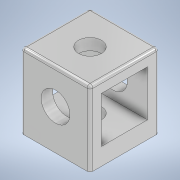
# Autodesk Inventor part: Kutup Aki
Saved by Autodesk Inventor 2021 (Build 250183000, 183)
## iProperties
Created: 2023-04-01
Part Number: Kutup Aki
Material: Iron, Cast
Document SubType Name: Modeling
Designer: user
Density: 7.15 g/cm^3
Appearance: Aluminum - Polished
Author: user
Autodesk Inventor part; units mm, degrees
ref_plane "YZ Plane" through (0, 0, 0) normal (1, 0, 0) x (0, 1, 0)
ref_plane "XZ Plane" through (0, 0, 0) normal (0, 1, 0) x (-1, 0, 0)
ref_plane "XY Plane" through (0, 0, 0) normal (0, 0, 1) x (1, 0, 0)
sketch "Sketch1" plane through (0, 0, 0) normal (0, 1, 0) x (-1, 0, 0)
  line L0 (6, -6) -> (-6, -6)
  line L1 (-6, -6) -> (-6, 6)
  line L2 (-6, 6) -> (6, 6)
  line L3 (6, 6) -> (6, -6)
  line L4 (6, -6) -> (-6, 6) construction
  line L5 (-6, -6) -> (6, 6) construction
  point P0 (0, 0)
  dimension "d0" = 12
  dimension "d1" = 12
  constraints: 12 end point, 2 midpoint, 2 parallel, 1 horizontal, 1 perpendicular
  measures "d0" distance of L1.end L2.end
  measures "d1" distance of L0.end L1.end
extrude "Extrusion1" add sketch "Sketch1" along normal blind 13
sketch "Sketch2" plane through (6, 0, 6) normal (1, 0, 0) x (0, 0, -1)
  line L0 (0, 0) -> (0, 13) projected
  line L1 (0, 13) -> (12, 13) projected
  line L2 (12, 13) -> (12, 0) projected
  line L3 (12, 0) -> (0, 0) projected
  line L4 (10, 11) -> (2, 11)
  line L5 (2, 11) -> (2, 2)
  line L6 (2, 2) -> (10, 2)
  line L7 (10, 2) -> (10, 11)
  line L8 (2, 11) -> (10, 11)
  line L9 (10, 11) -> (10, 3)
  line L10 (10, 3) -> (2, 3)
  line L11 (2, 3) -> (2, 11)
  point P0 (6, 0)
  dimension "d4" = 2
  dimension "d5" = 8
  dimension "d6" = 8
  constraints: 16 end point, 2 parallel, 1 horizontal, 1 perpendicular, 3 other
  measures "d4" distance between parallel lines of L1 L4
  measures "d5" distance of L9.end L10.end
  measures "d6" distance of L8.end L9.end
extrude "Extrusion2" cut sketch "Sketch2" against normal blind 13 contours L7 L10 L5 L4
sketch "Sketch3" plane through (-6, 0, 6) normal (0, 0, 1) x (1, 0, 0)
  line L0 (12, 13) -> (12, 0) projected
  line L1 (12, 0) -> (0, 0) projected
  line L2 (0, 0) -> (0, 13) projected
  line L3 (0, 13) -> (12, 13) projected
  line L4 (0, 13) -> (12, 13)
  line L5 (12, 13) -> (12, 1)
  line L6 (12, 1) -> (0, 1)
  line L7 (0, 1) -> (0, 13)
  line L8 (12, 13) -> (0, 1) construction
  line L9 (0, 13) -> (12, 13) construction
  line L10 (0, 13) -> (12, 1) construction
  circle A0 centre (6, 7) radius 2.5
  point P0 (6, 0)
  dimension "d9" = 12
  dimension "d10" = 12
  dimension "d11" = 5
  constraints: 12 end point, 2 parallel, 1 centre point, 1 horizontal, 1 midpoint, 1 perpendicular
  measures "d9" distance of L5.end L6.end
  measures "d10" distance of L4.end L5.end
  measures "d11" diameter of A0
extrude "Extrusion3" cut sketch "Sketch3" against normal blind 13 contours A0
sketch "Sketch4" plane through (0, 13, 0) normal (0, 1, 0) x (1, 0, 0)
  circle A0 centre (0, 0) radius 2
  dimension "d14" = 4
  constraints: 1 centre point, 1 coincident
  measures "d14" diameter of A0
extrude "Extrusion4" cut sketch "Sketch4" against normal blind 13
fillet "Fillet1" radius 0.5 8 edges at (0, 13, 6) (6, 6.5, 6) (-6, 6.5, 6) (-6, 6.5, -6) (6, 6.5, -6) (6, 13, 0) (0, 13, -6) (-6, 13, 0)
body "Solid1"
